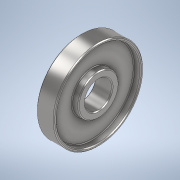
# Autodesk Inventor part: Колесо быстроходное
Saved by Autodesk Inventor 2021.2 (Build 252289000, 289)
## iProperties
Created: 2023-03-03
Part Number: Колесо быстроходное
Material: Сталь, углеродистая
Document SubType Name: Modeling
Designer: gdevc
Density: 7.85 g/cm^3
Appearance: С умеренной полировкой
Author: gdevc
Autodesk Inventor part; units mm, degrees
ref_plane "YZ Plane" through (0, 0, 0) normal (1, 0, 0) x (0, 1, 0)
ref_plane "XZ Plane" through (0, 0, 0) normal (0, 1, 0) x (-1, 0, 0)
ref_plane "XY Plane" through (0, 0, 0) normal (0, 0, 1) x (1, 0, 0)
sketch "Эскиз1" plane through (0, 0, 0) normal (0, 0, 1) x (1, 0, 0)
  line L0 (-31.7282, 0) -> (32.5604, 0) construction
  line L1 (-10, 15.5) -> (10, 15.5)
  line L2 (-10, 15.5) -> (-10, 23.25)
  line L3 (-10, 23.25) -> (10, 23.25)
  line L4 (10, 23.25) -> (10, 15.5)
  line L5 (-2.5, 23.25) -> (-2.5, 48)
  line L6 (-2.5, 48) -> (-10, 48)
  line L7 (-10, 48) -> (-10, 51.4)
  line L8 (0, 50.1433) -> (0, 23.25) construction
  line L9 (0, 23.25) -> (-2.5, 23.25)
  line L10 (2.5, 23.25) -> (2.5, 48)
  line L11 (2.5, 48) -> (10, 48)
  line L12 (10, 48) -> (10, 51.4)
  line L13 (-10, 51.4) -> (10, 51.4)
  point P0 (0, 0)
  point P1 (0, 15.5)
  dimension "d0" = 31
  dimension "d1" = 46.5
  dimension "d2" = 5
  dimension "d3" = 102.8
  dimension "d4" = 96
  dimension "d5" = 20
  dimension "d6" = 20
  constraints: 28 end point, 4 perpendicular, 4 symmetric about line, 3 horizontal, 2 midpoint, 2 point on line, 2 vertical, 1 collinear, 1 vertical alignment
  measures "d0" diameter of L1 L0
  measures "d1" diameter of L3 L0
  measures "d2" distance between parallel lines of L5 L10
  measures "d3" diameter of L13 L0
  measures "d4" diameter of L6 L0
  measures "d5" distance between parallel lines of L4 L2
  measures "d6" distance between parallel lines of L7 L12
revolve "Вращение1" add sketch "Эскиз1" angle 360 about axis through (-31.7282, 0, 0) along (1, 0, 0)
chamfer "Фаска1" distance 1 angle 45 8 edges at (-10, -51.4, 0) (-10, -48, 0) (-10, -23.25, 0) (-10, -15.5, 0) (10, -51.4, 0) (10, -48, 0) (10, -23.25, 0) (10, -15.5, 0)
fillet "Сопряжение1" radius 1 4 edges at (-2.5, -48, 0) (-2.5, -23.25, 0) (2.5, -48, 0) (2.5, -23.25, 0)
equation "\"d0\" = d"
equation "\"d1\" = d_ст"
equation "\"d2\" = C_колеса"
equation "\"d3\" = d_вершин"
equation "\"d\" = 31"
equation "\"d_ст\" = 1.5 * d"
equation "\"C_колеса\" = 5"
equation "\"d_вершин\" = 102.8"
